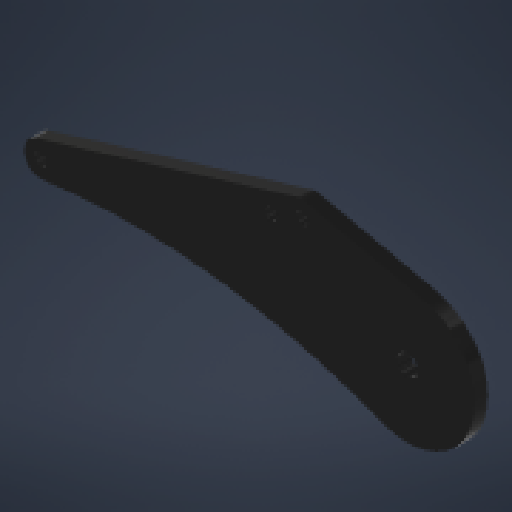
# Autodesk Inventor part: intakeside
Saved by Autodesk Inventor 2025.2 (Build 292293000, 293)
## iProperties
Created: 2026-01-05
Part Number: intakeside
Material: Acetal Resin, Black
Document SubType Name: Modeling
Designer: cloudy
Density: 1.425 g/cm^3
Appearance: Smooth - Black
Author: cloudy
Autodesk Inventor part; units mm, degrees
ref_plane "YZ Plane" through (0, 0, 0) normal (1, 0, 0) x (0, 1, 0)
ref_plane "XZ Plane" through (0, 0, 0) normal (0, 1, 0) x (-1, 0, 0)
ref_plane "XY Plane" through (0, 0, 0) normal (0, 0, 1) x (1, 0, 0)
sketch "Sketch1" plane through (0, 0, 0) normal (0, 0, 1) x (1, 0, 0)
  circle A0 centre (-98.962, -47.4274) radius 2.1844 projected
  circle A1 centre (39.6847, -45.4579) radius 2.9019 construction
  arc A2 (-100.8156, -41.354) -> (-98.7235, -53.773) centre (-98.962, -47.4274) ccw
  arc A3 (22.8757, -79.6496) -> (36.1943, -7.5182) centre (39.6847, -45.4579) ccw
  circle A4 centre (-11.8745, -21.7378) radius 6.35 construction
  arc A5 (-0.585, -10.9018) -> (-1.8569, -11.1517) centre (-0.0033, -17.2251) ccw
  line L0 (-11.8745, -21.7378) -> (-0.0033, -17.2251) construction
  line L1 (-98.962, -47.4274) -> (39.6847, -45.4579) construction
  circle A6 centre (-0.0033, -17.2251) radius 2.1844
  circle A7 centre (-11.8745, -21.7378) radius 2.1844
  line L2 (-100.8156, -41.354) -> (-1.8569, -11.1517)
  line L3 (36.1943, -7.5182) -> (-0.585, -10.9018)
  arc A8 (22.8757, -79.6496) -> (-98.7235, -53.773) centre (-89.1842, -307.5938) ccw
  circle A9 centre (39.6847, -45.4579) radius 4
  point P0 (0, 0)
  dimension "d0" = 12.7
  dimension "d1" = 76.2
  dimension "d2" = 12.7
  dimension "d3" = 20
  dimension "d4" = 4.3688
  dimension "d5" = 4.3688
  dimension "d6" = 254
  dimension "d7" = 8
  constraints: 8 centre point, 8 end point, 8 point on circle, 7 tangent, 5 coincident, 1 equal radius, 1 other
  measures "d0" diameter of A2
  measures "d1" diameter of A3
  measures "d2" diameter of A4
  measures "d3" angle of L1 L0
  measures "d4" diameter of A6
  measures "d5" diameter of A7
  measures "d6" radius of A8
  measures "d7" diameter of A9
extrude "Extrusion1" add sketch "Sketch1" along normal blind 5.08
body "Solid1"
